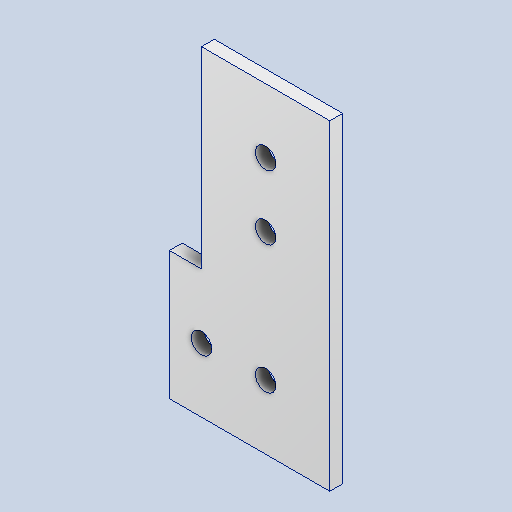
# Autodesk Inventor part: dribl-v3-Plate-6
Saved by Autodesk Inventor 2025.2 (Build 292293000, 293)
## iProperties
Created: 2025-04-05
Part Number: dribl-v3-Plate-6
Material: アルミニウム 6061
Document SubType Name: Modeling
Designer: haruy
Density: 2.7 g/cm^3
Appearance: アルミニウム - フラット
Author: haruy
Autodesk Inventor part; units mm, degrees
ref_plane "YZ Plane" through (0, 0, 0) normal (1, 0, 0) x (0, 1, 0)
ref_plane "XZ Plane" through (0, 0, 0) normal (0, 1, 0) x (-1, 0, 0)
ref_plane "XY Plane" through (0, 0, 0) normal (0, 0, 1) x (1, 0, 0)
derived "dribl-v3-Sketch-Base.ipt"
sketch "スケッチ6" plane through (250, -432.3334, -173) normal (0, 0, 1) x (1, 0, 0)
  line L0 (0, 0) -> (0, 200) projected
  line L1 (0, 30) -> (20, 30) projected
  line L2 (20, 0) -> (20, 200) projected
  line L3 (0, 0) -> (20, 0) projected
  circle A0 centre (10, 10) radius 1.6 projected
  circle A1 centre (10, 20) radius 1.6 projected
  line L4 (20, 201) -> (-320, 201) projected
  line L5 (-150, 201) -> (-150, 0) projected
  circle A2 centre (-310, 20) radius 1.6 projected
  circle A3 centre (-310, 10) radius 1.6 projected
  circle A4 centre (10, -10) radius 1.6 projected
  circle A5 centre (0, -10) radius 1.6 projected
  line L6 (20, 0) -> (-5, 0) projected
  line L7 (-5, 0) -> (-5, -20) projected
  line L8 (-5, -20) -> (20, -20) projected
  line L9 (20, -20) -> (20, 0) projected
  circle A6 centre (10, 180) radius 1.6 projected
  circle A7 centre (10, 190) radius 1.6 projected
  circle A8 centre (10, 210) radius 1.6 projected
  circle A9 centre (0, 210) radius 1.6 projected
  line L10 (20, 200) -> (-320, 200) projected
  line L11 (20, 220) -> (20, 200) projected
  line L12 (-320, 220) -> (20, 220) projected
  line L13 (0, 175) -> (20, 175) projected
  line L14 (-5, 220) -> (-5, 200) projected
  point P0 (-250, 432.3334)
extrude "押し出し1" add sketch "スケッチ6" along normal blind 2 contours L0 L1 L2 L3 | L3 L9 L8 L7 L6
